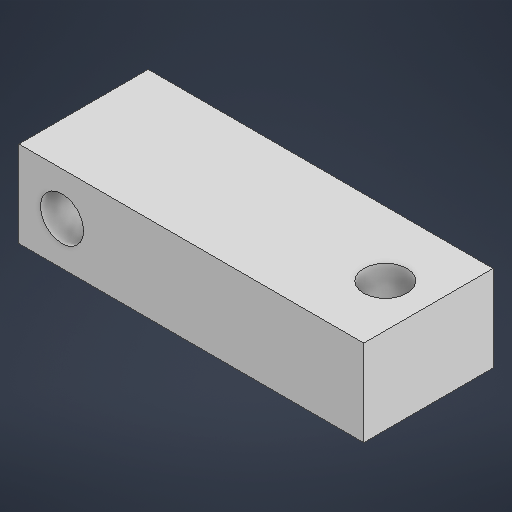
# Autodesk Inventor part: tie rod
Saved by Autodesk Inventor 2026.1 (Build 301233000, 233)
## iProperties
Created: 2026-06-10
Part Number: tie rod
Material: Generic
Document SubType Name: Modeling
Designer: share
Density: 1 g/cm^3
Appearance: Default
Author: share
Autodesk Inventor part; units mm, degrees
ref_plane "YZ Plane" through (0, 0, 0) normal (1, 0, 0) x (0, 1, 0)
ref_plane "XZ Plane" through (0, 0, 0) normal (0, 1, 0) x (-1, 0, 0)
ref_plane "XY Plane" through (0, 0, 0) normal (0, 0, 1) x (1, 0, 0)
sketch "Sketch1" plane through (0, 0, 0) normal (0, 1, 0) x (-1, 0, 0)
  line L0 (-50.8, -19.05) -> (50.8, -19.05)
  line L1 (50.8, -19.05) -> (50.8, 19.05)
  line L2 (50.8, 19.05) -> (-50.8, 19.05)
  line L3 (-50.8, 19.05) -> (-50.8, -19.05)
  line L4 (-50.8, -19.05) -> (50.8, 19.05) construction
  line L5 (50.8, -19.05) -> (-50.8, 19.05) construction
  point P0 (0, 0)
  dimension "d0" = 38.1
  dimension "d1" = 101.6
  constraints: 12 end point, 2 midpoint, 2 parallel, 1 horizontal, 1 perpendicular
  measures "d0" distance between parallel lines of L0 L2
  measures "d1" distance between parallel lines of L1 L3
extrude "Extrusion1" add sketch "Sketch1" along normal blind 25.4
sketch "Sketch2" plane through (50.8, 0, -19.05) normal (0, 0, -1) x (-1, 0, 0)
  line L0 (101.6, 0) -> (101.6, 25.4) projected
  line L1 (101.6, 12.7) -> (0, 12.7) construction
  line L2 (0, 0) -> (0, 25.4) projected
  circle A0 centre (88.9, 12.7) radius 6.35
  point P0 (50.8, 0)
  dimension "d4" = 12.7
  dimension "d5" = 12.7
  constraints: 2 end point, 2 midpoint, 1 centre point, 1 point on line
  measures "d4" distance from line of A0.centre L0
  measures "d5" diameter of A0
extrude "Extrusion2" cut sketch "Sketch2" against normal through all
sketch "Sketch3" plane through (0, 0, 0) normal (0, -1, 0) x (1, 0, 0)
  line L0 (50.8, 19.05) -> (50.8, -19.05) projected
  line L1 (50.8, 0) -> (-50.8, 0) construction
  line L2 (-50.8, -19.05) -> (-50.8, 19.05) projected
  circle A0 centre (38.1, 0) radius 6.35
  point P0 (0, 0)
  dimension "d8" = 12.7
  dimension "d9" = 12.7
  constraints: 2 end point, 2 midpoint, 1 centre point, 1 point on line
  measures "d8" distance from line of A0.centre L0
  measures "d9" diameter of A0
extrude "Extrusion3" cut sketch "Sketch3" against normal blind 25.4
body "Solid1"
